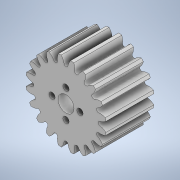
# Autodesk Inventor part: PINION
Saved by Autodesk Inventor 2021 (Build 250183000, 183)
## iProperties
Created: 2022-09-27
Part Number: PINION
Material: Generic
Document SubType Name: Modeling
Designer: ASUS
Density: 1 g/cm^3
Appearance: Default
Author: ASUS
Autodesk Inventor part; units mm, degrees
ref_plane "YZ Plane" through (0, 0, 0) normal (1, 0, 0) x (0, 1, 0)
ref_plane "XZ Plane" through (0, 0, 0) normal (0, 1, 0) x (-1, 0, 0)
ref_plane "XY Plane" through (0, 0, 0) normal (0, 0, 1) x (1, 0, 0)
sketch "Sketch1" plane through (0, 0, 0) normal (0, 0, 1) x (1, 0, 0)
  spline S0 degree 3 poles (-2.3918, 19.9824) (-2.3319, 19.9037) (-2.212, 19.7465) (-2.0415, 19.5038) (-1.8784, 19.2562) (-1.7238, 19.003) (-1.5786, 18.7444) (-1.4437, 18.4802) (-1.3205, 18.2104) (-1.2109, 17.9348) (-1.1332, 17.7) (-1.0819, 17.5091) (-1.0393, 17.3159) (-1.0179, 17.1189) (-0.97, 16.9268) (-0.9218, 16.7864) (-0.8588, 16.6519) (-0.7802, 16.5257) (-0.6986, 16.4324) (-0.6259, 16.3653) (-0.5659, 16.3216) (-0.5035, 16.2812) (-0.4363, 16.2497) (-0.3675, 16.2217) (-0.2954, 16.204) (-0.2225, 16.19) (-0.1235, 16.1859) (0, 16.1885) (0.1235, 16.1859) (0.2225, 16.19) (0.2954, 16.204) (0.3675, 16.2217) (0.4363, 16.2497) (0.5035, 16.2812) (0.5659, 16.3216) (0.6259, 16.3653) (0.6986, 16.4324) (0.7802, 16.5257) (0.8588, 16.6519) (0.9218, 16.7864) (0.97, 16.9268) (1.0179, 17.1189) (1.0393, 17.3159) (1.0819, 17.5091) (1.1332, 17.7) (1.2109, 17.9348) (1.3205, 18.2104) (1.4437, 18.4802) (1.5786, 18.7444) (1.7238, 19.003) (1.8784, 19.2562) (2.0415, 19.5038) (2.212, 19.7465) (2.3319, 19.9037) (2.3918, 19.9824) knots 0 0 0 0 0.029653 0.059306 0.088959 0.118612 0.148265 0.177917 0.207569 0.23722 0.266869 0.281695 0.29652 0.326167 0.340991 0.355815 0.370637 0.385456 0.400269 0.407684 0.415095 0.422509 0.429921 0.437334 0.444746 0.452159 0.45957 0.474397 0.489224 0.496635 0.504048 0.51146 0.518873 0.526285 0.533699 0.54111 0.548525 0.563338 0.578157 0.592978 0.607803 0.622627 0.652274 0.667099 0.681925 0.711574 0.741225 0.770877 0.800529 0.830182 0.859835 0.889488 0.919141 0.948794 0.948794 0.948794 0.948794
  circle A0 centre (0, 0) radius 16.1875 construction
  circle A1 centre (0, 0) radius 17.2669 construction
  circle A2 centre (0, 0) radius 18.375 construction
  circle A3 centre (0, 0) radius 20.125
  point P0 (-2.2136, 19.7454)
  point P1 (-2.0428, 19.503)
  point P2 (-1.8798, 19.2552)
  point P3 (-1.7254, 19.0021)
  point P4 (-1.5803, 18.7435)
  point P5 (-1.4456, 18.4793)
  point P6 (-1.3228, 18.2094)
  point P7 (-1.2136, 17.9337)
  point P8 (-1.1212, 17.652)
  point P9 (-1.083, 17.5088)
  point P10 (-1.0517, 17.3639)
  point P11 (-1.0037, 17.0713)
  point P12 (-0.968, 16.9274)
  point P13 (-0.9193, 16.7874)
  point P14 (-0.8562, 16.6533)
  point P15 (-0.777, 16.528)
  point P16 (-0.6798, 16.4163)
  point P17 (-0.6249, 16.3664)
  point P18 (-0.5655, 16.3221)
  point P19 (-0.5027, 16.2827)
  point P20 (-0.4361, 16.2503)
  point P21 (-0.367, 16.2234)
  point P22 (-0.2953, 16.2046)
  point P23 (-0.2223, 16.1918)
  point P24 (-0.1483, 16.1875)
  point P25 (0, 16.1875)
  point P26 (0.1483, 16.1875)
  point P27 (0.2223, 16.1918)
  point P28 (0.2953, 16.2046)
  point P29 (0.367, 16.2234)
  point P30 (0.4361, 16.2503)
  point P31 (0.5027, 16.2827)
  point P32 (0.5655, 16.3221)
  point P33 (0.6249, 16.3664)
  point P34 (0.6798, 16.4163)
  point P35 (0.777, 16.528)
  point P36 (0.8562, 16.6533)
  point P37 (0.9193, 16.7874)
  point P38 (0.968, 16.9274)
  point P39 (1.0037, 17.0713)
  point P40 (1.0517, 17.3639)
  point P41 (1.083, 17.5088)
  point P42 (1.1212, 17.652)
  point P43 (1.2136, 17.9337)
  point P44 (1.3228, 18.2094)
  point P45 (1.4456, 18.4793)
  point P46 (1.5803, 18.7435)
  point P47 (1.7254, 19.0021)
  point P48 (1.8798, 19.2552)
  point P49 (2.0428, 19.503)
  point P50 (2.2136, 19.7454)
  constraints: 4 centre point, 2 point on circle, 111 other
extrude "Extrusion1" add sketch "Sketch1" against normal blind 24
extrude "Extrusion2" cut sketch "Sketch1" against normal through all contours A3 S0 picked at (-0.3833, 18.8711)
pattern_circular "Circular Pattern1" count 20 over 360 about axis through (0, 0, -10) along (0, 0, 1) of "Extrusion2"
sketch "Sketch2" plane through (0, 0, 0) normal (0, 0, 1) x (1, 0, 0)
  circle A0 centre (0, 0) radius 4
  circle A1 centre (-7, 0) radius 1.55
  circle A2 centre (0, -7) radius 1.55
  circle A3 centre (7, 0) radius 1.55
  circle A4 centre (0, 7) radius 1.55
  dimension "d7" = 8
  dimension "d8" = 3.1
  dimension "d9" = 7
  dimension "d12" = 360
  constraints: 5 centre point, 1 coincident, 9 other
  measures "d7" diameter of A0
  measures "d8" diameter of A1
  measures "d9" distance of A1.centre point (0, 0)
extrude "Extrusion3" cut sketch "Sketch2" against normal through all
equation "\"d0\" = FaceWidth"
equation "\"Module\" = 1.75"
equation "\"PressureAngle\" = 20deg"
equation "\"UnitProfileClearance\" = 0.25"
equation "\"UnitRoundRadius\" = 0.35"
equation "\"HeadDiameter\" = 40.25"
equation "\"RootDiameter\" = 32.375"
equation "\"BaseDiameter\" = 34.5337"
equation "\"PitchDiameter\" = 36.75"
equation "\"FaceWidth\" = 24"
equation "\"HelixAngle\" = 0"
equation "\"UnitCorrection\" = 0"
equation "\"UnitAddendumModification\" = 0"
equation "\"CircularPitch\" = 5.497787"
equation "\"UnitBacklashShift\" = 0"
equation "\"TotalToolShift\" = 0"
equation "\"IsInternal\" = 0"
body "Solid1"
